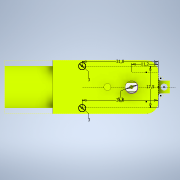
# Autodesk Inventor part: motor_placeholder
Saved by Autodesk Inventor 2021 (Build 250183000, 183)
## iProperties
Created: 2023-05-05
Part Number: motor_placeholder
Material: Generic
Document SubType Name: Modeling
Designer: assman
Density: 1 g/cm^3
Appearance: Default
Author: assman
Autodesk Inventor part; units mm, degrees
ref_plane "YZ Plane" through (0, 0, 0) normal (1, 0, 0) x (0, 1, 0)
ref_plane "XZ Plane" through (0, 0, 0) normal (0, 1, 0) x (-1, 0, 0)
ref_plane "XY Plane" through (0, 0, 0) normal (0, 0, 1) x (1, 0, 0)
sketch "Sketch1" plane through (0, 0, 0) normal (0, 1, 0) x (-1, 0, 0)
  line L0 (11.15, 32) -> (-11.15, 32)
  line L1 (-11.15, 32) -> (-11.15, -27)
  line L2 (11.15, -27) -> (11.15, 32)
  line L3 (11.15, 32) -> (-11.15, -32) construction
  line L4 (-11.15, 32) -> (11.15, -32) construction
  arc A0 (6.15, -32) -> (11.15, -27) centre (6.15, -27) ccw
  arc A1 (-11.15, -27) -> (-6.15, -32) centre (-6.15, -27) ccw
  line L5 (2.5547, -34.4) -> (0, -34.4) construction
  circle A2 centre (0, -34.4) radius 1.5
  line L6 (2.6003, -36.8) -> (-2.6003, -36.8)
  line L7 (-2.6003, -36.8) -> (-2.6003, -33)
  line L8 (2.5547, -32) -> (2.6003, -32)
  line L9 (2.6003, -33) -> (2.6003, -36.8)
  line L10 (2.6003, -36.8) -> (-2.6003, -32) construction
  line L11 (-2.6003, -36.8) -> (1.1023, -33.3826) construction
  line L12 (-6.15, -32) -> (-3.6003, -32)
  line L13 (3.6003, -32) -> (6.15, -32)
  arc A3 (3.6003, -32) -> (2.6003, -33) centre (3.6003, -33) ccw
  arc A4 (-2.6003, -33) -> (-3.6003, -32) centre (-3.6003, -33) ccw
  point P0 (0, 0)
  point P1 (0, -32)
  dimension "d19" = 3
  dimension "d14" = 22.3
  dimension "d15" = 64
  dimension "d16" = 5
  dimension "d17" = 5
  dimension "d18" = 2.4
  dimension "d20" = 1
  constraints: 28 end point, 10 tangent, 8 point on circle, 7 point on line, 5 parallel, 4 centre point, 3 horizontal, 3 midpoint, 2 perpendicular, 1 coincident, 1 equal radius, 3 other
  measures "d14" distance of L4.end L3.end
  measures "d15" distance of L3.end L0.end
  measures "d16" radius of A0
  measures "d17" radius of A1
  measures "d18" distance of L8.start L5.start
  measures "d20" radius of A3
extrude "Extrusion5" add sketch "Sketch1" along normal blind 18.7
sketch "Sketch5" plane through (0, 18.7, 0) normal (0, 1, 0) x (1, 0, 0)
  arc A0 (-6.15, 32) -> (-11.15, 27) centre (-6.15, 27) ccw construction
  line L0 (-11.15, 27) -> (-11.15, -32) construction
  line L1 (-11.15, -32) -> (11.15, -32) construction
  line L2 (11.15, -32) -> (11.15, 27) construction
  arc A1 (11.15, 27) -> (6.15, 32) centre (6.15, 27) ccw construction
  line L3 (6.15, 32) -> (3.6003, 32) construction
  arc A2 (3.6003, 32) -> (2.6003, 33) centre (3.6003, 33) ccw construction
  line L4 (2.6003, 33) -> (2.6003, 36.8) construction
  line L5 (2.6003, 36.8) -> (-2.6003, 36.8) construction
  line L6 (-2.6003, 36.8) -> (-2.6003, 33) construction
  arc A3 (-2.6003, 33) -> (-3.6003, 32) centre (-3.6003, 33) ccw construction
  line L7 (-3.6003, 32) -> (-6.15, 32) construction
  circle A4 centre (0, 34.4) radius 1.5 construction
  line L8 (-3.6003, 32) -> (-6.15, 32) construction
  line L9 (-6.15, 32) -> (-6.15, 20.8) construction
  circle A5 centre (0, 20.8) radius 2.6
  line L10 (0, 0) -> (0, 39.0389) construction
  line L11 (8.75, 32) -> (-8.75, 32) construction
  line L12 (-4.8752, 32) -> (4.8752, 32) construction
  line L13 (8.75, 32) -> (8.75, 0.2) construction
  circle A6 centre (8.75, 0.2) radius 1.5
  line L14 (-8.75, 32) -> (-8.75, 0.2) construction
  circle A7 centre (-8.75, 0.2) radius 1.5
  point P0 (0, 32)
  dimension "d23" = 11.2
  dimension "d24" = 5.2
  dimension "d29" = 17.5
  dimension "d30" = 31.8
  dimension "d31" = 3
  dimension "d32" = 31.8
  dimension "d33" = 3
  constraints: 18 end point, 8 centre point, 4 midpoint, 3 vertical, 2 coincident, 1 horizontal, 1 perpendicular
  measures "d23" distance of L7.end L9.end
  measures "d24" diameter of A5
  measures "d29" distance of L11.start L11.end
  measures "d30" distance of L11.start L13.end
  measures "d31" diameter of A6
  measures "d32" distance of L11.end L14.end
  measures "d33" diameter of A7
extrude "Extrusion6" cut sketch "Sketch5" against normal blind 18 contours A6 | A7
extrude "Extrusion7" add sketch "Sketch5" along normal blind 9.3 contours A5
sketch "Sketch6" plane through (0, 18.7, 0) normal (0, 1, 0) x (1, 0, 0)
  circle A0 centre (0, 20.8) radius 2.6 construction
  line L0 (0, 20.8) -> (0, 10.8) construction
  circle A1 centre (0, 10.8) radius 1.5
  point P0 (0, 0)
  dimension "d38" = 10
  dimension "d39" = 3
  constraints: 2 end point, 1 centre point, 1 coincident, 1 vertical
  measures "d38" distance of L0.start L0.end
  measures "d39" diameter of A1
extrude "Extrusion8" add sketch "Sketch6" along normal blind 2
sketch "Sketch7" plane through (0, 28, -20.8) normal (0, 1, 0) x (1, 0, 0)
  circle A0 centre (0, 0) radius 2.6 construction
  line L0 (1.8, -1.8762) -> (1.8, 1.8762)
  line L1 (-1.8, 1.8762) -> (-1.8, -1.8762)
  line L2 (-1.3648, -2.213) -> (1.3648, 2.213) construction
  line L3 (1.3648, -2.213) -> (-1.3648, 2.213) construction
  arc A1 (-1.8, 1.8762) -> (-1.8, -1.8762) centre (0, 0) ccw
  circle A2 centre (0, 0) radius 2.6 projected
  arc A3 (1.8, -1.8762) -> (1.8, 1.8762) centre (0, 0) ccw
  point P0 (0, -20.8)
  constraints: 8 end point, 4 point on circle, 2 centre point, 2 coincident, 2 midpoint, 1 parallel, 10 other
extrude "Extrusion9" cut sketch "Sketch7" against normal blind 8 contours L0 A2 | A1 L1
sketch "Sketch8" plane through (0, 28, 0) normal (0, 1, 0) x (1, 0, 0)
  line L0 (-1.8, 22.6762) -> (-1.8, 18.9238) construction
  arc A0 (-1.8, 18.9238) -> (1.8, 18.9238) centre (0, 20.8) ccw construction
  line L1 (1.8, 18.9238) -> (1.8, 22.6762) construction
  arc A1 (1.8, 22.6762) -> (-1.8, 22.6762) centre (0, 20.8) ccw construction
  circle A2 centre (0, 20.8) radius 0.75
  point P0 (0, 0)
  dimension "d45" = 1.5
  constraints: 1 centre point, 1 coincident
  measures "d45" diameter of A2
extrude "Extrusion10" cut sketch "Sketch8" against normal blind 8
sketch "Sketch9" plane through (-11.15, 0, 32) normal (0, 0, 1) x (1, 0, 0)
  line L0 (0, 0) -> (22.3, 0) construction
  line L1 (22.3, 0) -> (22.3, 18.7) construction
  line L2 (0, 18.7) -> (22.3, 18.7) construction
  line L3 (0, 0) -> (0, 18.7) construction
  circle A0 centre (11.15, 9.35) radius 8.75
  line L4 (0, 0) -> (0, 18.7) projected
  line L5 (0, 0) -> (22.3, 0)
  line L6 (22.3, 0) -> (22.3, 18.7)
  line L7 (22.3, 18.7) -> (0, 18.7)
  line L8 (0, 18.7) -> (0, 0)
  point P0 (11.15, 0)
  dimension "d48" = 17.5
  constraints: 8 end point, 2 parallel, 1 centre point, 1 horizontal, 1 perpendicular
  measures "d48" diameter of A0
extrude "Extrusion11" cut sketch "Sketch9" against normal blind 20
sketch "Sketch10" plane through (0, 0, 0) normal (0, -1, 0) x (1, 0, 0)
  line L0 (11.15, 12) -> (-11.15, 12) projected
  line L1 (-11.15, -27) -> (-11.15, 12) projected
  arc A0 (-11.15, -27) -> (-6.15, -32) centre (-6.15, -27) ccw projected
  line L2 (-3.6003, -32) -> (-6.15, -32) projected
  arc A1 (-2.6003, -33) -> (-3.6003, -32) centre (-3.6003, -33) ccw projected
  line L3 (-2.6003, -36.8) -> (-2.6003, -33) projected
  line L4 (2.6003, -36.8) -> (-2.6003, -36.8) projected
  line L5 (2.6003, -33) -> (2.6003, -36.8) projected
  arc A2 (3.6003, -32) -> (2.6003, -33) centre (3.6003, -33) ccw projected
  line L6 (6.15, -32) -> (3.6003, -32) projected
  arc A3 (6.15, -32) -> (11.15, -27) centre (6.15, -27) ccw projected
  line L7 (11.15, 12) -> (11.15, -27) projected
  circle A4 centre (0, -34.4) radius 1.5 projected
  arc A5 (-2.6003, -33) -> (-3.6003, -32) centre (-3.6003, -33) ccw projected
  line L8 (-3.6003, -32) -> (3.6003, -32)
  point P0 (0, 0)
  constraints: 2 end point, 1 collinear, 1 tangent
extrude "Extrusion12" cut sketch "Sketch10" against normal blind 5 contours A2 L5 L4 L3 A1 L8
sketch "Sketch11" plane through (0, 18.7, 0) normal (0, 1, 0) x (1, 0, 0)
  circle A0 centre (0, 34.4) radius 1.5 projected
  line L0 (-11.15, -12) -> (11.15, -12) projected
  line L1 (11.15, -12) -> (11.15, 27) projected
  arc A1 (11.15, 27) -> (6.15, 32) centre (6.15, 27) ccw projected
  line L2 (6.15, 32) -> (3.6003, 32) projected
  arc A2 (2.6003, 33) -> (3.6003, 32) centre (3.6003, 33) ccw projected
  line L3 (2.6003, 33) -> (2.6003, 36.8) projected
  line L4 (2.6003, 36.8) -> (-2.6003, 36.8) projected
  line L5 (-2.6003, 36.8) -> (-2.6003, 33) projected
  arc A3 (-3.6003, 32) -> (-2.6003, 33) centre (-3.6003, 33) ccw projected
  line L6 (-3.6003, 32) -> (-6.15, 32) projected
  arc A4 (-6.15, 32) -> (-11.15, 27) centre (-6.15, 27) ccw projected
  line L7 (-11.15, 27) -> (-11.15, -12) projected
  circle A5 centre (-8.75, 0.2) radius 1.5 projected
  circle A6 centre (8.75, 0.2) radius 1.5 projected
  circle A7 centre (0, 20.8) radius 2.6 projected
  circle A8 centre (0, 10.8) radius 1.5 projected
  arc A9 (-3.6003, 32) -> (-2.6003, 33) centre (-3.6003, 33) ccw projected
  line L8 (-3.6003, 32) -> (3.6003, 32)
  point P0 (0, 0)
  constraints: 2 end point, 1 collinear, 1 tangent
extrude "Extrusion13" cut sketch "Sketch11" against normal blind 5 contours A3 L5 L4 L3 A2 L8
body "Solid1"
body "Solid2"
